Autodesk Fusion 360 part; units mm, degrees
(part 14 of 18)
  line L8690 (7.8606, -38.6284) -> (8.6766, -38.6284)
  line L8691 (7.8606, -38.8324) -> (7.8606, -38.6284)
  line L8692 (25.2488, -38.6283) -> (24.4328, -38.6283)
  line L8693 (25.2488, -38.8324) -> (25.2488, -38.6283)
  line L8694 (24.4328, -38.6283) -> (24.4328, -38.8324)
  line L8695 (24.4328, -38.8324) -> (25.2488, -38.8324)
  line L8696 (27.4207, -38.0504) -> (27.4207, -39.4104)
  line L8697 (27.4207, -39.4104) -> (27.2167, -39.4104)
  line L8698 (27.2167, -39.4104) -> (27.2167, -38.0504)
  line L8699 (27.2167, -38.0504) -> (27.4207, -38.0504)
  line L8700 (27.7267, -38.8324) -> (26.9107, -38.8324)
  line L8701 (26.9107, -38.8324) -> (26.9107, -38.6284)
  line L8702 (26.9107, -38.6284) -> (27.7267, -38.6284)
  line L8703 (27.7267, -38.6284) -> (27.7267, -38.8324)
  line L8704 (24.4328, -19.5783) -> (24.4328, -19.7823)
  line L8705 (24.4328, -19.7823) -> (25.2488, -19.7823)
  line L8706 (25.2488, -19.5783) -> (24.4328, -19.5783)
  line L8707 (25.2488, -19.7823) -> (25.2488, -19.5783)
  line L8708 (27.4207, -20.3604) -> (27.2167, -20.3604)
  line L8709 (27.4207, -19.0003) -> (27.4207, -20.3604)
  line L8710 (27.2167, -20.3604) -> (27.2167, -19.0003)
  line L8711 (27.2167, -19.0003) -> (27.4207, -19.0003)
  line L8712 (27.7267, -19.7823) -> (26.9107, -19.7823)
  line L8713 (27.7267, -19.5783) -> (27.7267, -19.7823)
  line L8714 (26.9107, -19.7823) -> (26.9107, -19.5783)
  line L8715 (26.9107, -19.5783) -> (27.7267, -19.5783)
  line L8716 (25.2488, -57.6911) -> (24.4328, -57.6911)
  line L8717 (25.2488, -57.8951) -> (25.2488, -57.6911)
  line L8718 (24.4328, -57.6911) -> (24.4328, -57.8951)
  line L8719 (24.4328, -57.8951) -> (25.2488, -57.8951)
  line L8720 (27.4207, -58.4731) -> (27.2167, -58.4731)
  line L8721 (27.2167, -58.4731) -> (27.2167, -57.1131)
  line L8722 (27.2167, -57.1131) -> (27.4207, -57.1131)
  line L8723 (27.4207, -57.1131) -> (27.4207, -58.4731)
  line L8724 (27.7267, -57.6911) -> (27.7267, -57.8951)
  line L8725 (27.7267, -57.8951) -> (26.9107, -57.8951)
  line L8726 (26.9107, -57.6911) -> (27.7267, -57.6911)
  line L8727 (26.9107, -57.8951) -> (26.9107, -57.6911)
  line L8728 (44.2988, -19.5783) -> (43.4828, -19.5783)
  line L8729 (44.2988, -19.7823) -> (44.2988, -19.5783)
  line L8730 (43.4828, -19.5783) -> (43.4828, -19.7823)
  line L8731 (43.4828, -19.7823) -> (44.2988, -19.7823)
  line L8732 (46.2667, -20.3604) -> (46.2667, -19.0003)
  line L8733 (46.2667, -19.0003) -> (46.4707, -19.0003)
  line L8734 (46.4707, -19.0003) -> (46.4707, -20.3604)
  line L8735 (46.4707, -20.3604) -> (46.2667, -20.3604)
  line L8736 (46.7767, -19.5783) -> (46.7767, -19.7823)
  line L8737 (46.7767, -19.7823) -> (45.9607, -19.7823)
  line L8738 (45.9607, -19.7823) -> (45.9607, -19.5783)
  line L8739 (45.9607, -19.5783) -> (46.7767, -19.5783)
  line L8740 (43.4828, -57.6911) -> (43.4828, -57.8951)
  line L8741 (44.2988, -57.8951) -> (44.2988, -57.6911)
  line L8742 (44.2988, -57.6911) -> (43.4828, -57.6911)
  line L8743 (43.4828, -57.8951) -> (44.2988, -57.8951)
  line L8744 (46.4707, -57.1131) -> (46.4707, -58.4731)
  line L8745 (46.4707, -58.4731) -> (46.2667, -58.4731)
  line L8746 (46.2667, -58.4731) -> (46.2667, -57.1131)
  line L8747 (46.2667, -57.1131) -> (46.4707, -57.1131)
  line L8748 (45.9607, -57.6911) -> (46.7767, -57.6911)
  line L8749 (46.7767, -57.8951) -> (45.9607, -57.8951)
  line L8750 (45.9607, -57.8951) -> (45.9607, -57.6911)
  line L8751 (46.7767, -57.6911) -> (46.7767, -57.8951)
  line L8752 (43.4828, -38.6283) -> (43.4828, -38.8324)
  line L8753 (43.4828, -38.8324) -> (44.2988, -38.8324)
  line L8754 (44.2988, -38.8324) -> (44.2988, -38.6283)
  line L8755 (44.2988, -38.6283) -> (43.4828, -38.6283)
  line L8756 (46.4707, -39.4104) -> (46.2667, -39.4104)
  line L8757 (46.2667, -39.4104) -> (46.2667, -38.0504)
  line L8758 (46.4707, -38.0504) -> (46.4707, -39.4104)
  line L8759 (46.2667, -38.0504) -> (46.4707, -38.0504)
  line L8760 (45.9607, -38.8324) -> (45.9607, -38.6284)
  line L8761 (46.7767, -38.6284) -> (46.7767, -38.8324)
  line L8762 (45.9607, -38.6284) -> (46.7767, -38.6284)
  line L8763 (46.7767, -38.8324) -> (45.9607, -38.8324)
  line L8764 (214.9332, -19.5783) -> (214.9332, -19.7823)
  line L8765 (214.9332, -19.7823) -> (215.7492, -19.7823)
  line L8766 (215.7492, -19.7823) -> (215.7492, -19.5783)
  line L8767 (215.7492, -19.5783) -> (214.9332, -19.5783)
  line L8768 (217.9211, -19.0003) -> (217.9211, -20.3604)
  line L8769 (217.717, -20.3604) -> (217.717, -19.0003)
  line L8770 (217.9211, -20.3604) -> (217.717, -20.3604)
  line L8771 (217.717, -19.0003) -> (217.9211, -19.0003)
  line L8772 (217.411, -19.5783) -> (218.2271, -19.5783)
  line L8773 (218.2271, -19.5783) -> (218.2271, -19.7823)
  line L8774 (217.411, -19.7823) -> (217.411, -19.5783)
  line L8775 (218.2271, -19.7823) -> (217.411, -19.7823)
  line L8776 (214.9332, -76.9578) -> (215.7492, -76.9578)
  line L8777 (214.9332, -76.7538) -> (214.9332, -76.9578)
  line L8778 (215.7492, -76.7538) -> (214.9332, -76.7538)
  line L8779 (215.7492, -76.9578) -> (215.7492, -76.7538)
  line L8780 (217.717, -77.5359) -> (217.717, -76.1758)
  line L8781 (217.9211, -77.5359) -> (217.717, -77.5359)
  line L8782 (217.9211, -76.1758) -> (217.9211, -77.5359)
  line L8783 (217.717, -76.1758) -> (217.9211, -76.1758)
  line L8784 (217.411, -76.9579) -> (217.411, -76.7538)
  line L8785 (218.2271, -76.7538) -> (218.2271, -76.9579)
  line L8786 (218.2271, -76.9579) -> (217.411, -76.9579)
  line L8787 (217.411, -76.7538) -> (218.2271, -76.7538)
  line L8788 (215.7492, -57.8951) -> (215.7492, -57.6911)
  line L8789 (215.7492, -57.6911) -> (214.9332, -57.6911)
  line L8790 (214.9332, -57.8951) -> (215.7492, -57.8951)
  line L8791 (214.9332, -57.6911) -> (214.9332, -57.8951)
  line L8792 (217.717, -58.4731) -> (217.717, -57.1131)
  line L8793 (217.9211, -57.1131) -> (217.9211, -58.4731)
  line L8794 (217.717, -57.1131) -> (217.9211, -57.1131)
  line L8795 (217.9211, -58.4731) -> (217.717, -58.4731)
  line L8796 (218.2271, -57.6911) -> (218.2271, -57.8951)
  line L8797 (218.2271, -57.8951) -> (217.411, -57.8951)
  line L8798 (217.411, -57.6911) -> (218.2271, -57.6911)
  line L8799 (217.411, -57.8951) -> (217.411, -57.6911)
  line L8800 (214.9332, -38.8324) -> (215.7492, -38.8324)
  line L8801 (215.7492, -38.6283) -> (214.9332, -38.6283)
  line L8802 (215.7492, -38.8324) -> (215.7492, -38.6283)
  line L8803 (214.9332, -38.6283) -> (214.9332, -38.8324)
  line L8804 (217.717, -38.0504) -> (217.9211, -38.0504)
  line L8805 (217.9211, -39.4104) -> (217.717, -39.4104)
  line L8806 (217.717, -39.4104) -> (217.717, -38.0504)
  line L8807 (217.9211, -38.0504) -> (217.9211, -39.4104)
  line L8808 (217.411, -38.8324) -> (217.411, -38.6284)
  line L8809 (218.2271, -38.8324) -> (217.411, -38.8324)
  line L8810 (218.2271, -38.6284) -> (218.2271, -38.8324)
  line L8811 (217.411, -38.6284) -> (218.2271, -38.6284)
  line L8812 (196.6991, -38.6283) -> (195.8831, -38.6283)
  line L8813 (195.8831, -38.6283) -> (195.8831, -38.8324)
  line L8814 (196.6991, -38.8324) -> (196.6991, -38.6283)
  line L8815 (195.8831, -38.8324) -> (196.6991, -38.8324)
  line L8816 (198.871, -38.0504) -> (198.871, -39.4104)
  line L8817 (198.667, -39.4104) -> (198.667, -38.0504)
  line L8818 (198.667, -38.0504) -> (198.871, -38.0504)
  line L8819 (198.871, -39.4104) -> (198.667, -39.4104)
  line L8820 (199.177, -38.8324) -> (198.361, -38.8324)
  line L8821 (199.177, -38.6284) -> (199.177, -38.8324)
  line L8822 (198.361, -38.6284) -> (199.177, -38.6284)
  line L8823 (198.361, -38.8324) -> (198.361, -38.6284)
  line L8824 (195.8831, -76.9578) -> (196.6991, -76.9578)
  line L8825 (196.6991, -76.9578) -> (196.6991, -76.7538)
  line L8826 (195.8831, -76.7538) -> (195.8831, -76.9578)
  line L8827 (196.6991, -76.7538) -> (195.8831, -76.7538)
  line L8828 (198.667, -76.1758) -> (198.871, -76.1758)
  line L8829 (198.871, -77.5359) -> (198.667, -77.5359)
  line L8830 (198.871, -76.1758) -> (198.871, -77.5359)
  line L8831 (198.667, -77.5359) -> (198.667, -76.1758)
  line L8832 (198.361, -76.7538) -> (199.177, -76.7538)
  line L8833 (199.177, -76.7538) -> (199.177, -76.9579)
  line L8834 (198.361, -76.9579) -> (198.361, -76.7538)
  line L8835 (199.177, -76.9579) -> (198.361, -76.9579)
  line L8836 (195.8831, -57.6911) -> (195.8831, -57.8951)
  line L8837 (195.8831, -57.8951) -> (196.6991, -57.8951)
  line L8838 (196.6991, -57.6911) -> (195.8831, -57.6911)
  line L8839 (196.6991, -57.8951) -> (196.6991, -57.6911)
  line L8840 (198.667, -58.4731) -> (198.667, -57.1131)
  line L8841 (198.871, -58.4731) -> (198.667, -58.4731)
  line L8842 (198.667, -57.1131) -> (198.871, -57.1131)
  line L8843 (198.871, -57.1131) -> (198.871, -58.4731)
  line L8844 (199.177, -57.6911) -> (199.177, -57.8951)
  line L8845 (199.177, -57.8951) -> (198.361, -57.8951)
  line L8846 (198.361, -57.6911) -> (199.177, -57.6911)
  line L8847 (198.361, -57.8951) -> (198.361, -57.6911)
  line L8848 (196.6991, -19.5783) -> (195.8831, -19.5783)
  line L8849 (195.8831, -19.5783) -> (195.8831, -19.7823)
  line L8850 (195.8831, -19.7823) -> (196.6991, -19.7823)
  line L8851 (196.6991, -19.7823) -> (196.6991, -19.5783)
  line L8852 (198.667, -19.0003) -> (198.871, -19.0003)
  line L8853 (198.871, -19.0003) -> (198.871, -20.3604)
  line L8854 (198.667, -20.3604) -> (198.667, -19.0003)
  line L8855 (198.871, -20.3604) -> (198.667, -20.3604)
  line L8856 (199.177, -19.5783) -> (199.177, -19.7823)
  line L8857 (198.361, -19.7823) -> (198.361, -19.5783)
  line L8858 (198.361, -19.5783) -> (199.177, -19.5783)
  line L8859 (199.177, -19.7823) -> (198.361, -19.7823)
  arc A1894 (194.7833, -3.7496) -> (194.9835, -3.7496) centre (194.8834, -3.7496) ccw
  arc A1895 (194.9835, -3.7496) -> (194.7833, -3.7496) centre (194.8834, -3.7496) ccw
  line L8860 (190.2064, -3.5779) -> (190.2943, -3.79)
  line L8861 (190.2943, -4.89) -> (190.2064, -5.1021)
  line L8862 (190.2064, -5.1021) -> (189.9943, -5.19)
  line L8863 (189.6943, -3.79) -> (189.7822, -3.5779)
  line L8864 (190.2943, -3.79) -> (190.2943, -4.89)
  line L8865 (189.9943, -5.19) -> (189.7822, -5.1021)
  line L8866 (189.7822, -5.1021) -> (189.6943, -4.89)
  line L8867 (189.9943, -3.49) -> (190.2064, -3.5779)
  line L8868 (189.6943, -4.89) -> (189.6943, -3.79)
  line L8869 (189.7822, -3.5779) -> (189.9943, -3.49)
  line L8870 (181.3543, -3.49) -> (181.5664, -3.5778)
  line L8871 (181.0543, -3.79) -> (181.1421, -3.5778)
  line L8872 (181.0543, -4.89) -> (181.0543, -3.79)
  line L8873 (181.3543, -5.19) -> (181.1421, -5.1021)
  line L8874 (181.5664, -5.1021) -> (181.3543, -5.19)
  line L8875 (181.1421, -3.5778) -> (181.3543, -3.49)
  line L8876 (181.5664, -3.5778) -> (181.6543, -3.79)
  line L8877 (181.1421, -5.1021) -> (181.0543, -4.89)
  line L8878 (181.6543, -4.89) -> (181.5664, -5.1021)
  line L8879 (181.6543, -3.79) -> (181.6543, -4.89)
  line L8880 (189.7822, -0.8022) -> (189.6943, -0.5901)
  line L8881 (190.2064, -0.8022) -> (189.9943, -0.8901)
  line L8882 (190.2943, -0.5901) -> (190.2064, -0.8022)
  line L8883 (189.9943, 0.5099) -> (190.2064, 0.4221)
  line L8884 (190.2943, 0.2099) -> (190.2943, -0.5901)
  line L8885 (189.6943, 0.2099) -> (189.7822, 0.4221)
  line L8886 (189.9943, -0.8901) -> (189.7822, -0.8022)
  line L8887 (189.6943, -0.5901) -> (189.6943, 0.2099)
  line L8888 (190.2064, 0.4221) -> (190.2943, 0.2099)
  line L8889 (189.7822, 0.4221) -> (189.9943, 0.5099)
  line L8890 (181.5664, -0.8022) -> (181.3543, -0.8901)
  line L8891 (181.6543, 0.2099) -> (181.6543, -0.5901)
  line L8892 (181.1421, -0.8022) -> (181.0543, -0.5901)
  line L8893 (181.6543, -0.5901) -> (181.5664, -0.8022)
  line L8894 (181.0543, 0.2099) -> (181.1421, 0.4221)
  line L8895 (181.1421, 0.4221) -> (181.3543, 0.5099)
  line L8896 (181.3543, 0.5099) -> (181.5664, 0.4221)
  line L8897 (181.5664, 0.4221) -> (181.6543, 0.2099)
  line L8898 (181.0543, -0.5901) -> (181.0543, 0.2099)
  line L8899 (181.3543, -0.8901) -> (181.1421, -0.8022)
  arc A1896 (9.0131, -8.0011) -> (10.3131, -8.0011) centre (9.6631, -8.0011) ccw
  arc A1897 (10.3131, -8.0011) -> (9.0131, -8.0011) centre (9.6631, -8.0011) ccw
  arc A1898 (9.0131, -5.4611) -> (10.3131, -5.4611) centre (9.6631, -5.4611) ccw
  arc A1899 (10.3131, -5.4611) -> (9.0131, -5.4611) centre (9.6631, -5.4611) ccw
  arc A1900 (10.3131, -2.9211) -> (9.0131, -2.9211) centre (9.6631, -2.9211) ccw
  arc A1901 (9.0131, -2.9211) -> (10.3131, -2.9211) centre (9.6631, -2.9211) ccw
  arc A1902 (-5.4871, -8.0011) -> (-4.187, -8.0011) centre (-4.8371, -8.0011) ccw
  arc A1903 (-4.187, -8.0011) -> (-5.4871, -8.0011) centre (-4.8371, -8.0011) ccw
  arc A1904 (-5.4871, -2.9211) -> (-4.187, -2.9211) centre (-4.8371, -2.9211) ccw
  arc A1905 (-4.187, -2.9211) -> (-5.4871, -2.9211) centre (-4.8371, -2.9211) ccw
  line L8900 (3.4993, 0.5065) -> (3.6441, 0.2058)
  line L8901 (0.8266, 0.5065) -> (1.0875, 0.7146)
  line L8902 (1.0875, -0.6369) -> (0.8266, -0.4288)
  line L8903 (3.6441, -0.128) -> (3.4993, -0.4288)
  line L8904 (3.6441, 0.2058) -> (3.6441, -0.128)
  line L8905 (0.6817, -0.128) -> (0.6817, 0.2058)
  line L8906 (0.8266, -0.4288) -> (0.6817, -0.128)
  line L8907 (1.413, -0.7112) -> (1.0875, -0.6369)
  line L8908 (3.4993, -0.4288) -> (3.2383, -0.6369)
  line L8909 (1.0875, 0.7146) -> (1.413, 0.7889)
  line L8910 (3.2383, 0.7146) -> (3.4993, 0.5065)
  line L8911 (2.9129, -0.7112) -> (1.413, -0.7112)
  line L8912 (1.413, 0.7889) -> (2.9129, 0.7889)
  line L8913 (3.2383, -0.6369) -> (2.9129, -0.7112)
  line L8914 (0.6817, 0.2058) -> (0.8266, 0.5065)
  line L8915 (2.9129, 0.7889) -> (3.2383, 0.7146)
  line L8916 (1.0875, -10.2854) -> (1.413, -10.2111)
  line L8917 (3.6441, -11.128) -> (3.4993, -11.4288)
  line L8918 (1.413, -10.2111) -> (2.9129, -10.2111)
  line L8919 (1.413, -11.7112) -> (1.0875, -11.6369)
  line L8920 (1.0875, -11.6369) -> (0.8266, -11.4288)
  line L8921 (3.2383, -10.2854) -> (3.4993, -10.4935)
  line L8922 (3.6441, -10.7942) -> (3.6441, -11.128)
  line L8923 (0.8266, -11.4288) -> (0.6817, -11.128)
  line L8924 (0.6817, -11.128) -> (0.6817, -10.7942)
  line L8925 (3.4993, -10.4935) -> (3.6441, -10.7942)
  line L8926 (3.4993, -11.4288) -> (3.2383, -11.6369)
  line L8927 (3.2383, -11.6369) -> (2.9129, -11.7112)
  line L8928 (2.9129, -11.7112) -> (1.413, -11.7112)
  line L8929 (0.8266, -10.4935) -> (1.0875, -10.2854)
  line L8930 (2.9129, -10.2111) -> (3.2383, -10.2854)
  line L8931 (0.6817, -10.7942) -> (0.8266, -10.4935)
  arc A1906 (194.4974, -61.2644) -> (196.2974, -61.2644) centre (195.3974, -61.2644) ccw
  arc A1907 (196.2974, -61.2644) -> (194.4974, -61.2644) centre (195.3974, -61.2644) ccw
  arc A1908 (190.9974, -63.5184) -> (192.7974, -63.5184) centre (191.8974, -63.5184) ccw
  arc A1909 (192.7974, -63.5184) -> (190.9974, -63.5184) centre (191.8974, -63.5184) ccw
  arc A1910 (175.4474, -80.3272) -> (177.2474, -80.3272) centre (176.3474, -80.3272) ccw
  arc A1911 (177.2474, -80.3272) -> (175.4474, -80.3272) centre (176.3474, -80.3272) ccw
  arc A1912 (171.9473, -82.5812) -> (173.7473, -82.5812) centre (172.8473, -82.5812) ccw
  arc A1913 (173.7473, -82.5812) -> (171.9473, -82.5812) centre (172.8473, -82.5812) ccw
  arc A1914 (177.2474, -61.2644) -> (175.4474, -61.2644) centre (176.3474, -61.2644) ccw
  arc A1915 (175.4474, -61.2644) -> (177.2474, -61.2644) centre (176.3474, -61.2644) ccw
  arc A1916 (171.9473, -63.5184) -> (173.7473, -63.5184) centre (172.8473, -63.5184) ccw
  arc A1917 (173.7473, -63.5184) -> (171.9473, -63.5184) centre (172.8473, -63.5184) ccw
  arc A1918 (175.4474, -42.2017) -> (177.2474, -42.2017) centre (176.3474, -42.2017) ccw
  arc A1919 (177.2474, -42.2017) -> (175.4474, -42.2017) centre (176.3474, -42.2017) ccw
  arc A1920 (173.7473, -44.4557) -> (171.9473, -44.4557) centre (172.8473, -44.4557) ccw
  arc A1921 (171.9473, -44.4557) -> (173.7473, -44.4557) centre (172.8473, -44.4557) ccw
  arc A1922 (175.4474, -23.1516) -> (177.2474, -23.1516) centre (176.3474, -23.1516) ccw
  arc A1923 (177.2474, -23.1516) -> (175.4474, -23.1516) centre (176.3474, -23.1516) ccw
  arc A1924 (171.9473, -25.4057) -> (173.7473, -25.4057) centre (172.8473, -25.4057) ccw
  arc A1925 (173.7473, -25.4057) -> (171.9473, -25.4057) centre (172.8473, -25.4057) ccw
  arc A1926 (156.3973, -80.3272) -> (158.1973, -80.3272) centre (157.2973, -80.3272) ccw
  arc A1927 (158.1973, -80.3272) -> (156.3973, -80.3272) centre (157.2973, -80.3272) ccw
  arc A1928 (152.8973, -82.5812) -> (154.6973, -82.5812) centre (153.7973, -82.5812) ccw
  arc A1929 (154.6973, -82.5812) -> (152.8973, -82.5812) centre (153.7973, -82.5812) ccw
  arc A1930 (156.3973, -42.2017) -> (158.1973, -42.2017) centre (157.2973, -42.2017) ccw
  arc A1931 (158.1973, -42.2017) -> (156.3973, -42.2017) centre (157.2973, -42.2017) ccw
  arc A1932 (154.6973, -44.4557) -> (152.8973, -44.4557) centre (153.7973, -44.4557) ccw
  arc A1933 (152.8973, -44.4557) -> (154.6973, -44.4557) centre (153.7973, -44.4557) ccw
  arc A1934 (156.3973, -61.2644) -> (158.1973, -61.2644) centre (157.2973, -61.2644) ccw
  arc A1935 (158.1973, -61.2644) -> (156.3973, -61.2644) centre (157.2973, -61.2644) ccw
  arc A1936 (154.6973, -63.5184) -> (152.8973, -63.5184) centre (153.7973, -63.5184) ccw
  arc A1937 (152.8973, -63.5184) -> (154.6973, -63.5184) centre (153.7973, -63.5184) ccw
  arc A1938 (156.3973, -23.1516) -> (158.1973, -23.1516) centre (157.2973, -23.1516) ccw
  arc A1939 (158.1973, -23.1516) -> (156.3973, -23.1516) centre (157.2973, -23.1516) ccw
  arc A1940 (154.6973, -25.4057) -> (152.8973, -25.4057) centre (153.7973, -25.4057) ccw
  arc A1941 (152.8973, -25.4057) -> (154.6973, -25.4057) centre (153.7973, -25.4057) ccw
  arc A1942 (137.3473, -61.2644) -> (139.1473, -61.2644) centre (138.2473, -61.2644) ccw
  arc A1943 (139.1473, -61.2644) -> (137.3473, -61.2644) centre (138.2473, -61.2644) ccw
  arc A1944 (135.6473, -63.5184) -> (133.8473, -63.5184) centre (134.7473, -63.5184) ccw
  arc A1945 (133.8473, -63.5184) -> (135.6473, -63.5184) centre (134.7473, -63.5184) ccw
  arc A1946 (137.3473, -42.2017) -> (139.1473, -42.2017) centre (138.2473, -42.2017) ccw
  arc A1947 (139.1473, -42.2017) -> (137.3473, -42.2017) centre (138.2473, -42.2017) ccw
  arc A1948 (135.6473, -44.4557) -> (133.8473, -44.4557) centre (134.7473, -44.4557) ccw
  arc A1949 (133.8473, -44.4557) -> (135.6473, -44.4557) centre (134.7473, -44.4557) ccw
  arc A1950 (137.3473, -23.1516) -> (139.1473, -23.1516) centre (138.2473, -23.1516) ccw
  arc A1951 (139.1473, -23.1516) -> (137.3473, -23.1516) centre (138.2473, -23.1516) ccw
  arc A1952 (133.8473, -25.4057) -> (135.6473, -25.4057) centre (134.7473, -25.4057) ccw
  arc A1953 (135.6473, -25.4057) -> (133.8473, -25.4057) centre (134.7473, -25.4057) ccw
  arc A1954 (137.3473, -80.3272) -> (139.1473, -80.3272) centre (138.2473, -80.3272) ccw
  arc A1955 (139.1473, -80.3272) -> (137.3473, -80.3272) centre (138.2473, -80.3272) ccw
  arc A1956 (133.8473, -82.5812) -> (135.6473, -82.5812) centre (134.7473, -82.5812) ccw
  arc A1957 (135.6473, -82.5812) -> (133.8473, -82.5812) centre (134.7473, -82.5812) ccw
  arc A1958 (118.2972, -80.3272) -> (120.0972, -80.3272) centre (119.1972, -80.3272) ccw
  arc A1959 (120.0972, -80.3272) -> (118.2972, -80.3272) centre (119.1972, -80.3272) ccw
  arc A1960 (116.5972, -82.5812) -> (114.7972, -82.5812) centre (115.6972, -82.5812) ccw
  arc A1961 (114.7972, -82.5812) -> (116.5972, -82.5812) centre (115.6972, -82.5812) ccw
  arc A1962 (118.2972, -61.2644) -> (120.0972, -61.2644) centre (119.1972, -61.2644) ccw
  arc A1963 (120.0972, -61.2644) -> (118.2972, -61.2644) centre (119.1972, -61.2644) ccw
  arc A1964 (116.5972, -63.5184) -> (114.7972, -63.5184) centre (115.6972, -63.5184) ccw
  arc A1965 (114.7972, -63.5184) -> (116.5972, -63.5184) centre (115.6972, -63.5184) ccw
  arc A1966 (120.0972, -23.1516) -> (118.2972, -23.1516) centre (119.1972, -23.1516) ccw
  arc A1967 (118.2972, -23.1516) -> (120.0972, -23.1516) centre (119.1972, -23.1516) ccw
  arc A1968 (114.7972, -25.4057) -> (116.5972, -25.4057) centre (115.6972, -25.4057) ccw
  arc A1969 (116.5972, -25.4057) -> (114.7972, -25.4057) centre (115.6972, -25.4057) ccw
  arc A1970 (118.2972, -42.2017) -> (120.0972, -42.2017) centre (119.1972, -42.2017) ccw
  arc A1971 (120.0972, -42.2017) -> (118.2972, -42.2017) centre (119.1972, -42.2017) ccw
  arc A1972 (116.5972, -44.4557) -> (114.7972, -44.4557) centre (115.6972, -44.4557) ccw
  arc A1973 (114.7972, -44.4557) -> (116.5972, -44.4557) centre (115.6972, -44.4557) ccw
  arc A1974 (101.0472, -23.1516) -> (99.2472, -23.1516) centre (100.1472, -23.1516) ccw
  arc A1975 (99.2472, -23.1516) -> (101.0472, -23.1516) centre (100.1472, -23.1516) ccw
  arc A1976 (95.7472, -25.4057) -> (97.5472, -25.4057) centre (96.6472, -25.4057) ccw
  arc A1977 (97.5472, -25.4057) -> (95.7472, -25.4057) centre (96.6472, -25.4057) ccw
  arc A1978 (99.2472, -42.2017) -> (101.0472, -42.2017) centre (100.1472, -42.2017) ccw
  arc A1979 (101.0472, -42.2017) -> (99.2472, -42.2017) centre (100.1472, -42.2017) ccw
  arc A1980 (97.5472, -44.4557) -> (95.7472, -44.4557) centre (96.6472, -44.4557) ccw
  arc A1981 (95.7472, -44.4557) -> (97.5472, -44.4557) centre (96.6472, -44.4557) ccw
  arc A1982 (101.0472, -80.3272) -> (99.2472, -80.3272) centre (100.1472, -80.3272) ccw
  arc A1983 (99.2472, -80.3272) -> (101.0472, -80.3272) centre (100.1472, -80.3272) ccw
  arc A1984 (97.5472, -82.5812) -> (95.7472, -82.5812) centre (96.6472, -82.5812) ccw
  arc A1985 (95.7472, -82.5812) -> (97.5472, -82.5812) centre (96.6472, -82.5812) ccw
  arc A1986 (101.0472, -61.2644) -> (99.2472, -61.2644) centre (100.1472, -61.2644) ccw
  arc A1987 (99.2472, -61.2644) -> (101.0472, -61.2644) centre (100.1472, -61.2644) ccw
  arc A1988 (97.5472, -63.5184) -> (95.7472, -63.5184) centre (96.6472, -63.5184) ccw
  arc A1989 (95.7472, -63.5184) -> (97.5472, -63.5184) centre (96.6472, -63.5184) ccw
  arc A1990 (196.2974, -80.3272) -> (194.4974, -80.3272) centre (195.3974, -80.3272) ccw
  arc A1991 (194.4974, -80.3272) -> (196.2974, -80.3272) centre (195.3974, -80.3272) ccw
  arc A1992 (192.7974, -82.5812) -> (190.9974, -82.5812) centre (191.8974, -82.5812) ccw
  arc A1993 (190.9974, -82.5812) -> (192.7974, -82.5812) centre (191.8974, -82.5812) ccw
  arc A1994 (196.2974, -23.1516) -> (194.4974, -23.1516) centre (195.3974, -23.1516) ccw
  arc A1995 (194.4974, -23.1516) -> (196.2974, -23.1516) centre (195.3974, -23.1516) ccw
  arc A1996 (190.9974, -25.4057) -> (192.7974, -25.4057) centre (191.8974, -25.4057) ccw
  arc A1997 (192.7974, -25.4057) -> (190.9974, -25.4057) centre (191.8974, -25.4057) ccw
  arc A1998 (81.9972, -80.3272) -> (80.1972, -80.3272) centre (81.0972, -80.3272) ccw
  arc A1999 (80.1972, -80.3272) -> (81.9972, -80.3272) centre (81.0972, -80.3272) ccw
  arc A2000 (78.4972, -82.5812) -> (76.6972, -82.5812) centre (77.5972, -82.5812) ccw
  arc A2001 (76.6972, -82.5812) -> (78.4972, -82.5812) centre (77.5972, -82.5812) ccw
  arc A2002 (80.1972, -42.2017) -> (81.9972, -42.2017) centre (81.0972, -42.2017) ccw
  arc A2003 (81.9972, -42.2017) -> (80.1972, -42.2017) centre (81.0972, -42.2017) ccw
  arc A2004 (76.6972, -44.4557) -> (78.4972, -44.4557) centre (77.5972, -44.4557) ccw
  arc A2005 (78.4972, -44.4557) -> (76.6972, -44.4557) centre (77.5972, -44.4557) ccw
  arc A2006 (81.9972, -23.1516) -> (80.1972, -23.1516) centre (81.0972, -23.1516) ccw
  arc A2007 (80.1972, -23.1516) -> (81.9972, -23.1516) centre (81.0972, -23.1516) ccw
  arc A2008 (78.4972, -25.4057) -> (76.6972, -25.4057) centre (77.5972, -25.4057) ccw
  arc A2009 (76.6972, -25.4057) -> (78.4972, -25.4057) centre (77.5972, -25.4057) ccw
  arc A2010 (80.1972, -61.2644) -> (81.9972, -61.2644) centre (81.0972, -61.2644) ccw
  arc A2011 (81.9972, -61.2644) -> (80.1972, -61.2644) centre (81.0972, -61.2644) ccw
  arc A2012 (76.6972, -63.5184) -> (78.4972, -63.5184) centre (77.5972, -63.5184) ccw
  arc A2013 (78.4972, -63.5184) -> (76.6972, -63.5184) centre (77.5972, -63.5184) ccw
  arc A2014 (61.1471, -80.3272) -> (62.9471, -80.3272) centre (62.0471, -80.3272) ccw
  arc A2015 (62.9471, -80.3272) -> (61.1471, -80.3272) centre (62.0471, -80.3272) ccw
  arc A2016 (59.4471, -82.5812) -> (57.6471, -82.5812) centre (58.5471, -82.5812) ccw
  arc A2017 (57.6471, -82.5812) -> (59.4471, -82.5812) centre (58.5471, -82.5812) ccw
  arc A2018 (62.9471, -61.2644) -> (61.1471, -61.2644) centre (62.0471, -61.2644) ccw
  arc A2019 (61.1471, -61.2644) -> (62.9471, -61.2644) centre (62.0471, -61.2644) ccw
  arc A2020 (59.4471, -63.5184) -> (57.6471, -63.5184) centre (58.5471, -63.5184) ccw
  arc A2021 (57.6471, -63.5184) -> (59.4471, -63.5184) centre (58.5471, -63.5184) ccw
  arc A2022 (61.1471, -42.2017) -> (62.9471, -42.2017) centre (62.0471, -42.2017) ccw
  arc A2023 (62.9471, -42.2017) -> (61.1471, -42.2017) centre (62.0471, -42.2017) ccw
  arc A2024 (59.4471, -44.4557) -> (57.6471, -44.4557) centre (58.5471, -44.4557) ccw
  arc A2025 (57.6471, -44.4557) -> (59.4471, -44.4557) centre (58.5471, -44.4557) ccw
  arc A2026 (42.0971, -61.2644) -> (43.8971, -61.2644) centre (42.9971, -61.2644) ccw
  arc A2027 (43.8971, -61.2644) -> (42.0971, -61.2644) centre (42.9971, -61.2644) ccw
  arc A2028 (40.3971, -63.5184) -> (38.5971, -63.5184) centre (39.4971, -63.5184) ccw
  arc A2029 (38.5971, -63.5184) -> (40.3971, -63.5184) centre (39.4971, -63.5184) ccw
  arc A2030 (43.8971, -80.3272) -> (42.0971, -80.3272) centre (42.9971, -80.3272) ccw
  arc A2031 (42.0971, -80.3272) -> (43.8971, -80.3272) centre (42.9971, -80.3272) ccw
  arc A2032 (40.3971, -82.5812) -> (38.5971, -82.5812) centre (39.4971, -82.5812) ccw
  arc A2033 (38.5971, -82.5812) -> (40.3971, -82.5812) centre (39.4971, -82.5812) ccw
  arc A2034 (24.847, -80.3272) -> (23.047, -80.3272) centre (23.947, -80.3272) ccw
  arc A2035 (23.047, -80.3272) -> (24.847, -80.3272) centre (23.947, -80.3272) ccw
  arc A2036 (21.347, -82.5812) -> (19.547, -82.5812) centre (20.447, -82.5812) ccw
  arc A2037 (19.547, -82.5812) -> (21.347, -82.5812) centre (20.447, -82.5812) ccw
  arc A2038 (5.797, -80.3272) -> (3.997, -80.3272) centre (4.897, -80.3272) ccw
  arc A2039 (3.997, -80.3272) -> (5.797, -80.3272) centre (4.897, -80.3272) ccw
  arc A2040 (2.297, -82.5812) -> (0.497, -82.5812) centre (1.397, -82.5812) ccw
  arc A2041 (0.497, -82.5812) -> (2.297, -82.5812) centre (1.397, -82.5812) ccw
  arc A2042 (61.1471, -23.1516) -> (62.9471, -23.1516) centre (62.0471, -23.1516) ccw
  arc A2043 (62.9471, -23.1516) -> (61.1471, -23.1516) centre (62.0471, -23.1516) ccw
  arc A2044 (59.4471, -25.4057) -> (57.6471, -25.4057) centre (58.5471, -25.4057) ccw
  arc A2045 (57.6471, -25.4057) -> (59.4471, -25.4057) centre (58.5471, -25.4057) ccw
  arc A2046 (42.0971, -42.2017) -> (43.8971, -42.2017) centre (42.9971, -42.2017) ccw
  arc A2047 (43.8971, -42.2017) -> (42.0971, -42.2017) centre (42.9971, -42.2017) ccw
  arc A2048 (40.3971, -44.4557) -> (38.5971, -44.4557) centre (39.4971, -44.4557) ccw
  arc A2049 (38.5971, -44.4557) -> (40.3971, -44.4557) centre (39.4971, -44.4557) ccw
  arc A2050 (43.8971, -23.1516) -> (42.0971, -23.1516) centre (42.9971, -23.1516) ccw
  arc A2051 (42.0971, -23.1516) -> (43.8971, -23.1516) centre (42.9971, -23.1516) ccw
  arc A2052 (38.5971, -25.4057) -> (40.3971, -25.4057) centre (39.4971, -25.4057) ccw
  arc A2053 (40.3971, -25.4057) -> (38.5971, -25.4057) centre (39.4971, -25.4057) ccw
  arc A2054 (24.847, -23.1516) -> (23.047, -23.1516) centre (23.947, -23.1516) ccw
  arc A2055 (23.047, -23.1516) -> (24.847, -23.1516) centre (23.947, -23.1516) ccw
  arc A2056 (19.547, -25.4057) -> (21.347, -25.4057) centre (20.447, -25.4057) ccw
  arc A2057 (21.347, -25.4057) -> (19.547, -25.4057) centre (20.447, -25.4057) ccw
  arc A2058 (24.847, -61.2644) -> (23.047, -61.2644) centre (23.947, -61.2644) ccw
  arc A2059 (23.047, -61.2644) -> (24.847, -61.2644) centre (23.947, -61.2644) ccw
  arc A2060 (21.347, -63.5184) -> (19.547, -63.5184) centre (20.447, -63.5184) ccw
  arc A2061 (19.547, -63.5184) -> (21.347, -63.5184) centre (20.447, -63.5184) ccw
  arc A2062 (23.047, -42.2017) -> (24.847, -42.2017) centre (23.947, -42.2017) ccw
  arc A2063 (24.847, -42.2017) -> (23.047, -42.2017) centre (23.947, -42.2017) ccw
  arc A2064 (21.347, -44.4557) -> (19.547, -44.4557) centre (20.447, -44.4557) ccw
  arc A2065 (19.547, -44.4557) -> (21.347, -44.4557) centre (20.447, -44.4557) ccw
  arc A2066 (3.997, -23.1516) -> (5.797, -23.1516) centre (4.897, -23.1516) ccw
  arc A2067 (5.797, -23.1516) -> (3.997, -23.1516) centre (4.897, -23.1516) ccw
  arc A2068 (0.497, -25.4057) -> (2.297, -25.4057) centre (1.397, -25.4057) ccw
  arc A2069 (2.297, -25.4057) -> (0.497, -25.4057) centre (1.397, -25.4057) ccw
  arc A2070 (5.797, -42.2017) -> (3.997, -42.2017) centre (4.897, -42.2017) ccw
  arc A2071 (3.997, -42.2017) -> (5.797, -42.2017) centre (4.897, -42.2017) ccw
  arc A2072 (2.297, -44.4557) -> (0.497, -44.4557) centre (1.397, -44.4557) ccw
  arc A2073 (0.497, -44.4557) -> (2.297, -44.4557) centre (1.397, -44.4557) ccw
  arc A2074 (5.797, -61.2644) -> (3.997, -61.2644) centre (4.897, -61.2644) ccw
  arc A2075 (3.997, -61.2644) -> (5.797, -61.2644) centre (4.897, -61.2644) ccw
  arc A2076 (2.297, -63.5184) -> (0.497, -63.5184) centre (1.397, -63.5184) ccw
  arc A2077 (0.497, -63.5184) -> (2.297, -63.5184) centre (1.397, -63.5184) ccw
  arc A2078 (215.3474, -61.2644) -> (213.5474, -61.2644) centre (214.4474, -61.2644) ccw
  arc A2079 (213.5474, -61.2644) -> (215.3474, -61.2644) centre (214.4474, -61.2644) ccw
  arc A2080 (210.0474, -63.5184) -> (211.8474, -63.5184) centre (210.9474, -63.5184) ccw
  arc A2081 (211.8474, -63.5184) -> (210.0474, -63.5184) centre (210.9474, -63.5184) ccw
  arc A2082 (213.5474, -42.2017) -> (215.3474, -42.2017) centre (214.4474, -42.2017) ccw
  arc A2083 (215.3474, -42.2017) -> (213.5474, -42.2017) centre (214.4474, -42.2017) ccw
  arc A2084 (210.0474, -44.4557) -> (211.8474, -44.4557) centre (210.9474, -44.4557) ccw
  arc A2085 (211.8474, -44.4557) -> (210.0474, -44.4557) centre (210.9474, -44.4557) ccw
  arc A2086 (213.5474, -23.1516) -> (215.3474, -23.1516) centre (214.4474, -23.1516) ccw
  arc A2087 (215.3474, -23.1516) -> (213.5474, -23.1516) centre (214.4474, -23.1516) ccw
  arc A2088 (211.8474, -25.4057) -> (210.0474, -25.4057) centre (210.9474, -25.4057) ccw
  arc A2089 (210.0474, -25.4057) -> (211.8474, -25.4057) centre (210.9474, -25.4057) ccw
  arc A2090 (215.3474, -80.3272) -> (213.5474, -80.3272) centre (214.4474, -80.3272) ccw
  arc A2091 (213.5474, -80.3272) -> (215.3474, -80.3272) centre (214.4474, -80.3272) ccw
  arc A2092 (211.8474, -82.5812) -> (210.0474, -82.5812) centre (210.9474, -82.5812) ccw
  arc A2093 (210.0474, -82.5812) -> (211.8474, -82.5812) centre (210.9474, -82.5812) ccw
  arc A2094 (194.4974, -42.2017) -> (196.2974, -42.2017) centre (195.3974, -42.2017) ccw
  arc A2095 (196.2974, -42.2017) -> (194.4974, -42.2017) centre (195.3974, -42.2017) ccw
  arc A2096 (192.7974, -44.4557) -> (190.9974, -44.4557) centre (191.8974, -44.4557) ccw
  arc A2097 (190.9974, -44.4557) -> (192.7974, -44.4557) centre (191.8974, -44.4557) ccw
  arc A2098 (176.6224, -4.318) -> (175.4224, -4.318) centre (176.0224, -4.318) ccw
  arc A2099 (175.4224, -4.318) -> (176.6224, -4.318) centre (176.0224, -4.318) ccw
  arc A2100 (174.0823, -4.318) -> (172.8823, -4.318) centre (173.4823, -4.318) ccw
  arc A2101 (172.8823, -4.318) -> (174.0823, -4.318) centre (173.4823, -4.318) ccw
  arc A2102 (202.5909, -11.075) -> (202.2859, -11.075) centre (202.4384, -11.075) ccw
  arc A2103 (202.2859, -11.075) -> (202.5909, -11.075) centre (202.4384, -11.075) ccw
  arc A2104 (200.2539, -9.83) -> (200.5589, -9.83) centre (200.4064, -9.83) ccw
  arc A2105 (200.5589, -9.83) -> (200.2539, -9.83) centre (200.4064, -9.83) ccw
  arc A2106 (201.5749, -10.414) -> (201.2699, -10.414) centre (201.4224, -10.414) ccw
  arc A2107 (201.2699, -10.414) -> (201.5749, -10.414) centre (201.4224, -10.414) ccw
  arc A2108 (199.0276, -9.144) -> (199.3326, -9.144) centre (199.1801, -9.144) ccw
  arc A2109 (199.3326, -9.144) -> (199.0276, -9.144) centre (199.1801, -9.144) ccw
  arc A2110 (203.8609, -11.659) -> (203.5559, -11.659) centre (203.7084, -11.659) ccw
  arc A2111 (203.5559, -11.659) -> (203.8609, -11.659) centre (203.7084, -11.659) ccw
  arc A2112 (205.4609, -12.243) -> (205.1559, -12.243) centre (205.3084, -12.243) ccw
  arc A2113 (205.1559, -12.243) -> (205.4609, -12.243) centre (205.3084, -12.243) ccw
  arc A2114 (198.0949, -8.56) -> (198.3999, -8.56) centre (198.2474, -8.56) ccw
  arc A2115 (198.3999, -8.56) -> (198.0949, -8.56) centre (198.2474, -8.56) ccw
  arc A2116 (190.077, -6.6518) -> (189.772, -6.6518) centre (189.9245, -6.6518) ccw
  arc A2117 (189.772, -6.6518) -> (190.077, -6.6518) centre (189.9245, -6.6518) ccw
  arc A2118 (203.7181, -5.1015) -> (204.0231, -5.1015) centre (203.8706, -5.1015) ccw
  arc A2119 (204.0231, -5.1015) -> (203.7181, -5.1015) centre (203.8706, -5.1015) ccw
  arc A2120 (200.1621, -4.5935) -> (200.4671, -4.5935) centre (200.3146, -4.5935) ccw
  arc A2121 (200.4671, -4.5935) -> (200.1621, -4.5935) centre (200.3146, -4.5935) ccw
  arc A2122 (213.5675, -7.3628) -> (213.8725, -7.3628) centre (213.72, -7.3628) ccw
  arc A2123 (213.8725, -7.3628) -> (213.5675, -7.3628) centre (213.72, -7.3628) ccw
  arc A2124 (197.6164, -7.1088) -> (197.3114, -7.1088) centre (197.4639, -7.1088) ccw
  arc A2125 (197.3114, -7.1088) -> (197.6164, -7.1088) centre (197.4639, -7.1088) ccw
  arc A2126 (208.0519, -4.953) -> (207.7469, -4.953) centre (207.8994, -4.953) ccw
  arc A2127 (207.7469, -4.953) -> (208.0519, -4.953) centre (207.8994, -4.953) ccw
  arc A2128 (202.2859, -6.35) -> (202.5909, -6.35) centre (202.4384, -6.35) ccw
  arc A2129 (202.5909, -6.35) -> (202.2859, -6.35) centre (202.4384, -6.35) ccw
  arc A2130 (194.2089, -5.588) -> (193.9039, -5.588) centre (194.0564, -5.588) ccw
  arc A2131 (193.9039, -5.588) -> (194.2089, -5.588) centre (194.0564, -5.588) ccw
  arc A2132 (173.7618, -2.032) -> (173.4568, -2.032) centre (173.6093, -2.032) ccw
  arc A2133 (173.4568, -2.032) -> (173.7618, -2.032) centre (173.6093, -2.032) ccw
  arc A2134 (176.0479, -1.27) -> (175.7429, -1.27) centre (175.8954, -1.27) ccw
  arc A2135 (175.7429, -1.27) -> (176.0479, -1.27) centre (175.8954, -1.27) ccw
  arc A2136 (197.5109, -1.194) -> (197.2059, -1.194) centre (197.3584, -1.194) ccw
  arc A2137 (197.2059, -1.194) -> (197.5109, -1.194) centre (197.3584, -1.194) ccw
  arc A2138 (197.7139, -0.381) -> (198.0189, -0.381) centre (197.8664, -0.381) ccw
  arc A2139 (198.0189, -0.381) -> (197.7139, -0.381) centre (197.8664, -0.381) ccw
  arc A2140 (200.0509, -3.048) -> (199.7459, -3.048) centre (199.8984, -3.048) ccw
  arc A2141 (199.7459, -3.048) -> (200.0509, -3.048) centre (199.8984, -3.048) ccw
  arc A2142 (207.1629, -13.462) -> (206.8579, -13.462) centre (207.0104, -13.462) ccw
  arc A2143 (206.8579, -13.462) -> (207.1629, -13.462) centre (207.0104, -13.462) ccw
  arc A2144 (191.0978, -6.668) -> (191.4028, -6.668) centre (191.2503, -6.668) ccw
  arc A2145 (191.4028, -6.668) -> (191.0978, -6.668) centre (191.2503, -6.668) ccw
  arc A2146 (198.8439, -0.262) -> (198.5389, -0.262) centre (198.6914, -0.262) ccw
  arc A2147 (198.5389, -0.262) -> (198.8439, -0.262) centre (198.6914, -0.262) ccw
  arc A2148 (205.7019, -2.532) -> (205.3969, -2.532) centre (205.5494, -2.532) ccw
  arc A2149 (205.3969, -2.532) -> (205.7019, -2.532) centre (205.5494, -2.532) ccw
  arc A2150 (202.3999, -1.262) -> (202.0949, -1.262) centre (202.2474, -1.262) ccw
  arc A2151 (202.0949, -1.262) -> (202.3999, -1.262) centre (202.2474, -1.262) ccw
  arc A2152 (198.6649, -6.5507) -> (198.9699, -6.5507) centre (198.8174, -6.5507) ccw
  arc A2153 (198.9699, -6.5507) -> (198.6649, -6.5507) centre (198.8174, -6.5507) ccw
  arc A2154 (213.3135, -6.3468) -> (213.6185, -6.3468) centre (213.466, -6.3468) ccw
  arc A2155 (213.6185, -6.3468) -> (213.3135, -6.3468) centre (213.466, -6.3468) ccw
  arc A2156 (197.6084, -7.9089) -> (197.9134, -7.9089) centre (197.7609, -7.9089) ccw
  arc A2157 (197.9134, -7.9089) -> (197.6084, -7.9089) centre (197.7609, -7.9089) ccw
  arc A2158 (207.1979, -14.2026) -> (207.5029, -14.2026) centre (207.3504, -14.2026) ccw
  arc A2159 (207.5029, -14.2026) -> (207.1979, -14.2026) centre (207.3504, -14.2026) ccw
  arc A2160 (210.9542, -15.3914) -> (210.6492, -15.3914) centre (210.8017, -15.3914) ccw
  arc A2161 (210.6492, -15.3914) -> (210.9542, -15.3914) centre (210.8017, -15.3914) ccw
  arc A2162 (208.2764, -8.563) -> (208.5814, -8.563) centre (208.4289, -8.563) ccw
  arc A2163 (208.5814, -8.563) -> (208.2764, -8.563) centre (208.4289, -8.563) ccw
  arc A2164 (208.5814, -9.3628) -> (208.2764, -9.3628) centre (208.4289, -9.3628) ccw
  arc A2165 (208.2764, -9.3628) -> (208.5814, -9.3628) centre (208.4289, -9.3628) ccw
  arc A2166 (89.1501, -21.4469) -> (89.4551, -21.4469) centre (89.3026, -21.4469) ccw
  arc A2167 (89.4551, -21.4469) -> (89.1501, -21.4469) centre (89.3026, -21.4469) ccw
  arc A2168 (208.5814, -10.1629) -> (208.2764, -10.1629) centre (208.4289, -10.1629) ccw
  arc A2169 (208.2764, -10.1629) -> (208.5814, -10.1629) centre (208.4289, -10.1629) ccw
  arc A2170 (206.2954, -12.7598) -> (205.9904, -12.7598) centre (206.1429, -12.7598) ccw
  arc A2171 (205.9904, -12.7598) -> (206.2954, -12.7598) centre (206.1429, -12.7598) ccw
  arc A2172 (205.3959, -4.0861) -> (205.7009, -4.0861) centre (205.5484, -4.0861) ccw
  arc A2173 (205.7009, -4.0861) -> (205.3959, -4.0861) centre (205.5484, -4.0861) ccw
  arc A2174 (208.6979, -2.3081) -> (209.0029, -2.3081) centre (208.8504, -2.3081) ccw
  arc A2175 (209.0029, -2.3081) -> (208.6979, -2.3081) centre (208.8504, -2.3081) ccw
  arc A2176 (210.284, -14.0756) -> (210.589, -14.0756) centre (210.4365, -14.0756) ccw
  arc A2177 (210.589, -14.0756) -> (210.284, -14.0756) centre (210.4365, -14.0756) ccw
  arc A2178 (213.002, -16.4886) -> (212.697, -16.4886) centre (212.8495, -16.4886) ccw
  arc A2179 (212.697, -16.4886) -> (213.002, -16.4886) centre (212.8495, -16.4886) ccw
  arc A2180 (214.6211, -16.2346) -> (214.9261, -16.2346) centre (214.7736, -16.2346) ccw
  arc A2181 (214.9261, -16.2346) -> (214.6211, -16.2346) centre (214.7736, -16.2346) ccw
  arc A2182 (211.522, -14.3296) -> (211.827, -14.3296) centre (211.6745, -14.3296) ccw
  arc A2183 (211.827, -14.3296) -> (211.522, -14.3296) centre (211.6745, -14.3296) ccw
  arc A2184 (215.7439, -41.8179) -> (216.0489, -41.8179) centre (215.8964, -41.8179) ccw
  arc A2185 (216.0489, -41.8179) -> (215.7439, -41.8179) centre (215.8964, -41.8179) ccw
  arc A2186 (213.4971, -11.1546) -> (213.1921, -11.1546) centre (213.3446, -11.1546) ccw
  arc A2187 (213.1921, -11.1546) -> (213.4971, -11.1546) centre (213.3446, -11.1546) ccw
  arc A2188 (216.6465, -59.3385) -> (216.9515, -59.3385) centre (216.799, -59.3385) ccw
  arc A2189 (216.9515, -59.3385) -> (216.6465, -59.3385) centre (216.799, -59.3385) ccw
  arc A2190 (217.5769, -13) -> (217.2719, -13) centre (217.4244, -13) ccw
  arc A2191 (217.2719, -13) -> (217.5769, -13) centre (217.4244, -13) ccw
  arc A2192 (217.2719, -15.113) -> (217.5769, -15.113) centre (217.4244, -15.113) ccw
  arc A2193 (217.5769, -15.113) -> (217.2719, -15.113) centre (217.4244, -15.113) ccw
  arc A2194 (210.8459, -13.1866) -> (210.5409, -13.1866) centre (210.6934, -13.1866) ccw
  arc A2195 (210.5409, -13.1866) -> (210.8459, -13.1866) centre (210.6934, -13.1866) ccw
  arc A2196 (195.4657, -2.8941) -> (195.1607, -2.8941) centre (195.3132, -2.8941) ccw
  arc A2197 (195.1607, -2.8941) -> (195.4657, -2.8941) centre (195.3132, -2.8941) ccw
  arc A2198 (216.0019, -11.557) -> (216.3069, -11.557) centre (216.1544, -11.557) ccw
  arc A2199 (216.3069, -11.557) -> (216.0019, -11.557) centre (216.1544, -11.557) ccw
  arc A2200 (211.9221, -8.7631) -> (212.2269, -8.7631) centre (212.0745, -8.7631) ccw
  arc A2201 (212.2269, -8.7631) -> (211.9221, -8.7631) centre (212.0745, -8.7631) ccw
  arc A2202 (211.9221, -7.7631) -> (212.2269, -7.7631) centre (212.0745, -7.7631) ccw
  arc A2203 (212.2269, -7.7631) -> (211.9221, -7.7631) centre (212.0745, -7.7631) ccw
  arc A2204 (209.9224, -8.7629) -> (210.2272, -8.7629) centre (210.0748, -8.7629) ccw
  arc A2205 (210.2272, -8.7629) -> (209.9224, -8.7629) centre (210.0748, -8.7629) ccw
  arc A2206 (209.9224, -7.7631) -> (210.2272, -7.7631) centre (210.0748, -7.7631) ccw
  arc A2207 (210.2272, -7.7631) -> (209.9224, -7.7631) centre (210.0748, -7.7631) ccw
  arc A2208 (211.9221, -9.7631) -> (212.2269, -9.7631) centre (212.0745, -9.7631) ccw
  arc A2209 (212.2269, -9.7631) -> (211.9221, -9.7631) centre (212.0745, -9.7631) ccw
  arc A2210 (209.9221, -9.7631) -> (210.2269, -9.7631) centre (210.0745, -9.7631) ccw
  arc A2211 (210.2269, -9.7631) -> (209.9221, -9.7631) centre (210.0745, -9.7631) ccw
  arc A2212 (211.2269, -8.7631) -> (210.9221, -8.7631) centre (211.0745, -8.7631) ccw
  arc A2213 (210.9221, -8.7631) -> (211.2269, -8.7631) centre (211.0745, -8.7631) ccw
  arc A2214 (211.2275, -9.7626) -> (210.9227, -9.7626) centre (211.0751, -9.7626) ccw
  arc A2215 (210.9227, -9.7626) -> (211.2275, -9.7626) centre (211.0751, -9.7626) ccw
  arc A2216 (210.9221, -7.7631) -> (211.2269, -7.7631) centre (211.0745, -7.7631) ccw
  arc A2217 (211.2269, -7.7631) -> (210.9221, -7.7631) centre (211.0745, -7.7631) ccw
  arc A2218 (201.4005, -1.505) -> (201.5205, -1.505) centre (201.4605, -1.505) ccw
  arc A2219 (201.5205, -1.505) -> (201.4005, -1.505) centre (201.4605, -1.505) ccw
  arc A2220 (207.5145, -5.263) -> (207.6344, -5.263) centre (207.5744, -5.263) ccw
  arc A2221 (207.6344, -5.263) -> (207.5145, -5.263) centre (207.5744, -5.263) ccw
  arc A2222 (186.9662, -7.1311) -> (186.8463, -7.1311) centre (186.9063, -7.1311) ccw
  arc A2223 (186.8463, -7.1311) -> (186.9662, -7.1311) centre (186.9063, -7.1311) ccw
  arc A2224 (183.9944, -6.331) -> (183.8745, -6.331) centre (183.9345, -6.331) ccw
  arc A2225 (183.8745, -6.331) -> (183.9944, -6.331) centre (183.9345, -6.331) ccw
  arc A2226 (212.5755, -3.786) -> (212.6955, -3.786) centre (212.6355, -3.786) ccw
  arc A2227 (212.6955, -3.786) -> (212.5755, -3.786) centre (212.6355, -3.786) ccw
  arc A2228 (138.3754, -77.7107) -> (138.4953, -77.7107) centre (138.4354, -77.7107) ccw
  arc A2229 (138.4953, -77.7107) -> (138.3754, -77.7107) centre (138.4354, -77.7107) ccw
  arc A2230 (138.4953, -20.5352) -> (138.3754, -20.5352) centre (138.4354, -20.5352) ccw
  arc A2231 (138.3754, -20.5352) -> (138.4953, -20.5352) centre (138.4354, -20.5352) ccw
  arc A2232 (138.3754, -39.5852) -> (138.4953, -39.5852) centre (138.4354, -39.5852) ccw
  arc A2233 (138.4953, -39.5852) -> (138.3754, -39.5852) centre (138.4354, -39.5852) ccw
  arc A2234 (138.3754, -58.648) -> (138.4953, -58.648) centre (138.4354, -58.648) ccw
  arc A2235 (138.4953, -58.648) -> (138.3754, -58.648) centre (138.4354, -58.648) ccw
  arc A2236 (157.4254, -20.5352) -> (157.5454, -20.5352) centre (157.4854, -20.5352) ccw
  arc A2237 (157.5454, -20.5352) -> (157.4254, -20.5352) centre (157.4854, -20.5352) ccw
  arc A2238 (157.5454, -77.7107) -> (157.4254, -77.7107) centre (157.4854, -77.7107) ccw
  arc A2239 (157.4254, -77.7107) -> (157.5454, -77.7107) centre (157.4854, -77.7107) ccw
  arc A2240 (157.4254, -58.648) -> (157.5454, -58.648) centre (157.4854, -58.648) ccw
  arc A2241 (157.5454, -58.648) -> (157.4254, -58.648) centre (157.4854, -58.648) ccw
  arc A2242 (157.5454, -39.5852) -> (157.4254, -39.5852) centre (157.4854, -39.5852) ccw
  arc A2243 (157.4254, -39.5852) -> (157.5454, -39.5852) centre (157.4854, -39.5852) ccw
  arc A2244 (176.4755, -20.5352) -> (176.5954, -20.5352) centre (176.5354, -20.5352) ccw
  arc A2245 (176.5954, -20.5352) -> (176.4755, -20.5352) centre (176.5354, -20.5352) ccw
  arc A2246 (176.4755, -77.7107) -> (176.5954, -77.7107) centre (176.5354, -77.7107) ccw
  arc A2247 (176.5954, -77.7107) -> (176.4755, -77.7107) centre (176.5354, -77.7107) ccw
  arc A2248 (176.4755, -58.648) -> (176.5954, -58.648) centre (176.5354, -58.648) ccw
  arc A2249 (176.5954, -58.648) -> (176.4755, -58.648) centre (176.5354, -58.648) ccw
  arc A2250 (176.4755, -39.5852) -> (176.5954, -39.5852) centre (176.5354, -39.5852) ccw
  arc A2251 (176.5954, -39.5852) -> (176.4755, -39.5852) centre (176.5354, -39.5852) ccw
  arc A2252 (100.3953, -77.7107) -> (100.2753, -77.7107) centre (100.3353, -77.7107) ccw
  arc A2253 (100.2753, -77.7107) -> (100.3953, -77.7107) centre (100.3353, -77.7107) ccw
  arc A2254 (100.3953, -58.648) -> (100.2753, -58.648) centre (100.3353, -58.648) ccw
  arc A2255 (100.2753, -58.648) -> (100.3953, -58.648) centre (100.3353, -58.648) ccw
  arc A2256 (100.2753, -20.5352) -> (100.3953, -20.5352) centre (100.3353, -20.5352) ccw
  arc A2257 (100.3953, -20.5352) -> (100.2753, -20.5352) centre (100.3353, -20.5352) ccw
  arc A2258 (100.3953, -39.5852) -> (100.2753, -39.5852) centre (100.3353, -39.5852) ccw
  arc A2259 (100.2753, -39.5852) -> (100.3953, -39.5852) centre (100.3353, -39.5852) ccw
  arc A2260 (119.4453, -20.5352) -> (119.3253, -20.5352) centre (119.3853, -20.5352) ccw
  arc A2261 (119.3253, -20.5352) -> (119.4453, -20.5352) centre (119.3853, -20.5352) ccw
  arc A2262 (119.3253, -58.648) -> (119.4453, -58.648) centre (119.3853, -58.648) ccw
  arc A2263 (119.4453, -58.648) -> (119.3253, -58.648) centre (119.3853, -58.648) ccw
  arc A2264 (119.4453, -39.5852) -> (119.3253, -39.5852) centre (119.3853, -39.5852) ccw
  arc A2265 (119.3253, -39.5852) -> (119.4453, -39.5852) centre (119.3853, -39.5852) ccw
  arc A2266 (119.3253, -77.7107) -> (119.4453, -77.7107) centre (119.3853, -77.7107) ccw
  arc A2267 (119.4453, -77.7107) -> (119.3253, -77.7107) centre (119.3853, -77.7107) ccw
  arc A2268 (5.0251, -77.7107) -> (5.1451, -77.7107) centre (5.0851, -77.7107) ccw
  arc A2269 (5.1451, -77.7107) -> (5.0251, -77.7107) centre (5.0851, -77.7107) ccw
  arc A2270 (24.1951, -77.7107) -> (24.0752, -77.7107) centre (24.1351, -77.7107) ccw
  arc A2271 (24.0752, -77.7107) -> (24.1951, -77.7107) centre (24.1351, -77.7107) ccw
  arc A2272 (43.1252, -77.7107) -> (43.2451, -77.7107) centre (43.1852, -77.7107) ccw
  arc A2273 (43.2451, -77.7107) -> (43.1252, -77.7107) centre (43.1852, -77.7107) ccw
  arc A2274 (62.2952, -20.5352) -> (62.1752, -20.5352) centre (62.2352, -20.5352) ccw
  arc A2275 (62.1752, -20.5352) -> (62.2952, -20.5352) centre (62.2352, -20.5352) ccw
  arc A2276 (62.2952, -77.7107) -> (62.1752, -77.7107) centre (62.2352, -77.7107) ccw
  arc A2277 (62.1752, -77.7107) -> (62.2952, -77.7107) centre (62.2352, -77.7107) ccw
  arc A2278 (62.1752, -39.5852) -> (62.2952, -39.5852) centre (62.2352, -39.5852) ccw
  arc A2279 (62.2952, -39.5852) -> (62.1752, -39.5852) centre (62.2352, -39.5852) ccw
  arc A2280 (62.1752, -58.648) -> (62.2952, -58.648) centre (62.2352, -58.648) ccw
  arc A2281 (62.2952, -58.648) -> (62.1752, -58.648) centre (62.2352, -58.648) ccw
  arc A2282 (81.2253, -39.5852) -> (81.3452, -39.5852) centre (81.2852, -39.5852) ccw
  arc A2283 (81.3452, -39.5852) -> (81.2253, -39.5852) centre (81.2852, -39.5852) ccw
  arc A2284 (81.2253, -77.7107) -> (81.3452, -77.7107) centre (81.2852, -77.7107) ccw
  arc A2285 (81.3452, -77.7107) -> (81.2253, -77.7107) centre (81.2852, -77.7107) ccw
  arc A2286 (81.2253, -20.5352) -> (81.3452, -20.5352) centre (81.2852, -20.5352) ccw
  arc A2287 (81.3452, -20.5352) -> (81.2253, -20.5352) centre (81.2852, -20.5352) ccw
  arc A2288 (81.2253, -58.648) -> (81.3452, -58.648) centre (81.2852, -58.648) ccw
  arc A2289 (81.3452, -58.648) -> (81.2253, -58.648) centre (81.2852, -58.648) ccw
  arc A2290 (5.1451, -58.648) -> (5.0251, -58.648) centre (5.0851, -58.648) ccw
  arc A2291 (5.0251, -58.648) -> (5.1451, -58.648) centre (5.0851, -58.648) ccw
  arc A2292 (5.1451, -20.5352) -> (5.0251, -20.5352) centre (5.0851, -20.5352) ccw
  arc A2293 (5.0251, -20.5352) -> (5.1451, -20.5352) centre (5.0851, -20.5352) ccw
  arc A2294 (5.1451, -39.5852) -> (5.0251, -39.5852) centre (5.0851, -39.5852) ccw
  arc A2295 (5.0251, -39.5852) -> (5.1451, -39.5852) centre (5.0851, -39.5852) ccw
  arc A2296 (24.0752, -39.5852) -> (24.1951, -39.5852) centre (24.1351, -39.5852) ccw
  arc A2297 (24.1951, -39.5852) -> (24.0752, -39.5852) centre (24.1351, -39.5852) ccw
  arc A2298 (24.1951, -20.5352) -> (24.0752, -20.5352) centre (24.1351, -20.5352) ccw
  arc A2299 (24.0752, -20.5352) -> (24.1951, -20.5352) centre (24.1351, -20.5352) ccw
  arc A2300 (24.1951, -58.648) -> (24.0752, -58.648) centre (24.1351, -58.648) ccw
  arc A2301 (24.0752, -58.648) -> (24.1951, -58.648) centre (24.1351, -58.648) ccw
  arc A2302 (43.1252, -20.5352) -> (43.2451, -20.5352) centre (43.1852, -20.5352) ccw
  arc A2303 (43.2451, -20.5352) -> (43.1252, -20.5352) centre (43.1852, -20.5352) ccw
  arc A2304 (43.1252, -58.648) -> (43.2451, -58.648) centre (43.1852, -58.648) ccw
  arc A2305 (43.2451, -58.648) -> (43.1252, -58.648) centre (43.1852, -58.648) ccw
  arc A2306 (43.2451, -39.5852) -> (43.1252, -39.5852) centre (43.1852, -39.5852) ccw
  arc A2307 (43.1252, -39.5852) -> (43.2451, -39.5852) centre (43.1852, -39.5852) ccw
  arc A2308 (214.6955, -20.5352) -> (214.5755, -20.5352) centre (214.6355, -20.5352) ccw
  arc A2309 (214.5755, -20.5352) -> (214.6955, -20.5352) centre (214.6355, -20.5352) ccw
  arc A2310 (214.5755, -77.7107) -> (214.6955, -77.7107) centre (214.6355, -77.7107) ccw
  arc A2311 (214.6955, -77.7107) -> (214.5755, -77.7107) centre (214.6355, -77.7107) ccw
  arc A2312 (214.5755, -58.648) -> (214.6955, -58.648) centre (214.6355, -58.648) ccw
  arc A2313 (214.6955, -58.648) -> (214.5755, -58.648) centre (214.6355, -58.648) ccw
  arc A2314 (214.5755, -39.5852) -> (214.6955, -39.5852) centre (214.6355, -39.5852) ccw
  arc A2315 (214.6955, -39.5852) -> (214.5755, -39.5852) centre (214.6355, -39.5852) ccw
  arc A2316 (195.5255, -39.5852) -> (195.6454, -39.5852) centre (195.5855, -39.5852) ccw